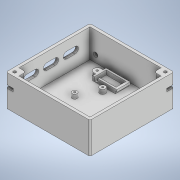
# Autodesk Inventor part: caixa transmissao
Saved by Autodesk Inventor 2022 (Build 260153000, 153)
## iProperties
Created: 2022-03-12
Part Number: caixa transmissao
Material: Genérico
Document SubType Name: Modeling
Designer: Hanter
Density: 1 g/cm^3
Appearance: Padrão
Author: Hanter
Autodesk Inventor part; units mm, degrees
ref_plane "YZ Plane" through (0, 0, 0) normal (1, 0, 0) x (0, 1, 0)
ref_plane "XZ Plane" through (0, 0, 0) normal (0, 1, 0) x (-1, 0, 0)
ref_plane "XY Plane" through (0, 0, 0) normal (0, 0, 1) x (1, 0, 0)
sketch "Esboço1" plane through (0, 0, 0) normal (0, 1, 0) x (-1, 0, 0)
  line L0 (-55, 55) -> (55, 55)
  line L1 (55, 55) -> (55, -55)
  line L2 (55, -55) -> (-55, -55)
  line L3 (-55, -55) -> (-55, 55)
  line L4 (-55, 55) -> (55, -55) construction
  line L5 (55, 55) -> (-55, -55) construction
  point P0 (0, 0)
  dimension "d0" = 110
  dimension "d1" = 110
  constraints: 12 end point, 2 midpoint, 2 parallel, 1 horizontal, 1 perpendicular
  measures "d0" distance of L1.end L2.end
  measures "d1" distance of L0.end L1.end
extrude "Extrusão1" add sketch "Esboço1" along normal blind 3 and the other way blind 1
sketch "Esboço2" plane through (0, 3, 0) normal (0, 1, 0) x (1, 0, 0)
  line L0 (47, -47) -> (-9.07, -47)
  line L1 (47, 26.73) -> (47, -47)
  line L2 (55, -55) -> (55, 55) projected
  line L3 (-55, -55) -> (55, -55) projected
  circle A0 centre (44.23, -44.26) radius 1.35
  circle A1 centre (44.23, 24.32) radius 1.35
  circle A2 centre (-6.57, -44.26) radius 1.35
  circle A3 centre (-6.57, 24.32) radius 1.35
  circle A4 centre (-6.57, -44.26) radius 4
  circle A5 centre (-6.57, 24.32) radius 4
  circle A6 centre (44.23, 24.32) radius 4
  circle A7 centre (44.23, -44.26) radius 4
  point P0 (0, 0)
  dimension "d8" = 2.7
  dimension "d13" = 68.58
  dimension "d16" = 50.8
  dimension "d21" = 8
  dimension "d22" = 8
  dimension "d23" = 8
  dimension "d24" = 8
  constraints: 8 centre point, 4 coincident, 4 end point, 2 horizontal, 1 vertical, 6 other
  measures "d8" diameter of A0
  measures "d13" distance of A0.centre A1.centre
  measures "d16" distance of A0.centre A2.centre
  measures "d21" diameter of A4
  measures "d22" diameter of A5
  measures "d23" diameter of A6
  measures "d24" diameter of A7
extrude "Extrusão2" add sketch "Esboço2" along normal blind 6
sketch "Esboço3" plane through (0, 3, 0) normal (0, 1, 0) x (1, 0, 0)
  line L0 (47, -47) -> (-9.07, -47)
  line L1 (-9.07, -47) -> (-9.07, 26.73)
  line L2 (-9.07, 26.73) -> (47, 26.73)
  line L3 (47, 26.73) -> (47, -47)
  line L4 (55, -55) -> (55, 55) projected
  line L5 (-55, -55) -> (55, -55) projected
  line L6 (55, 55) -> (-55, 55) projected
  line L7 (-55, -55) -> (-55, 55) projected
  circle A0 centre (-36.1, -31.5) radius 1.4
  circle A1 centre (-20.1, -1.5) radius 1.4
  circle A2 centre (-36.1, -31.5) radius 3.5
  circle A3 centre (-20.1, -1.5) radius 3.5
  point P0 (0, 0)
  dimension "d27" = 56.07
  dimension "d28" = 73.73
  dimension "d29" = 8
  dimension "d30" = 8
  dimension "d42" = 2.8
  dimension "d43" = 2.8
  dimension "d49" = 7
  dimension "d50" = 7
  constraints: 8 end point, 4 centre point, 2 coincident, 2 parallel, 1 horizontal, 1 perpendicular
  measures "d27" distance of L1.end L2.end
  measures "d28" distance of L0.end L1.end
  measures "d29" distance between parallel lines of L4 L3
  measures "d30" distance between parallel lines of L5 L0
  measures "d42" diameter of A0
  measures "d43" diameter of A1
  measures "d49" diameter of A2
  measures "d50" diameter of A3
extrude "Extrusão3" add sketch "Esboço3" along normal blind 6 contours A2 | A3
sketch "Esboço4" plane through (0, 3, 0) normal (0, 1, 0) x (1, 0, 0)
  line L0 (47, -47) -> (-9.07, -47)
  line L1 (-9.07, -47) -> (-9.07, 26.73)
  line L2 (-9.07, 26.73) -> (47, 26.73)
  line L3 (47, 26.73) -> (47, -47)
  line L4 (55, -55) -> (55, 55) projected
  line L5 (-55, -55) -> (55, -55) projected
  line L6 (-38.6, -38) -> (-17.6, -38)
  line L7 (-17.6, -38) -> (-17.6, 5)
  line L8 (-17.6, 5) -> (-38.6, 5)
  line L9 (-38.6, 5) -> (-38.6, -38)
  line L10 (-55, 55) -> (-55, -55) projected
  line L11 (3, 47.7) -> (-25, 47.7)
  line L12 (-25, 47.7) -> (-25, 33.7)
  line L13 (-25, 33.7) -> (3, 33.7)
  line L14 (3, 33.7) -> (3, 47.7)
  line L15 (55, 55) -> (-55, 55) projected
  line L16 (-27.5, 31.2) -> (6.5, 31.2)
  line L17 (6.5, 31.2) -> (6.5, 50.2)
  line L18 (6.5, 50.2) -> (-27.5, 50.2)
  line L19 (-27.5, 50.2) -> (-27.5, 31.2)
  line L20 (-27.5, 35.7) -> (-35.5, 35.7)
  line L21 (-35.5, 35.7) -> (-35.5, 45.7)
  line L22 (-35.5, 45.7) -> (-27.5, 45.7)
  line L23 (-27.5, 45.7) -> (-27.5, 35.7)
  point P0 (0, 0)
  dimension "d53" = 56.07
  dimension "d54" = 73.73
  dimension "d55" = 8
  dimension "d56" = 8
  dimension "d57" = 21
  dimension "d58" = 43
  dimension "d59" = 16.4
  dimension "d60" = 17
  dimension "d64" = 52
  dimension "d65" = 14
  dimension "d66" = 28
  dimension "d67" = 2.5
  dimension "d68" = 2.5
  dimension "d69" = 2.5
  dimension "d70" = 3.5
  dimension "d71" = 8
  dimension "d81" = 2
  dimension "d82" = 2
  constraints: 40 end point, 10 parallel, 5 horizontal, 5 perpendicular, 1 point on line
  measures "d53" distance of L1.end L2.end
  measures "d54" distance of L0.end L1.end
  measures "d55" distance between parallel lines of L4 L3
  measures "d56" distance between parallel lines of L5 L0
  measures "d57" distance of L8.end L7.end
  measures "d58" distance of L7.end L6.end
  measures "d59" distance between parallel lines of L10 L9
  measures "d60" distance between parallel lines of L5 L6
  measures "d64" distance between parallel lines of L4 L14
  measures "d65" distance of L11.end L12.end
  measures "d66" distance of L11.start L11.end
  measures "d67" distance between parallel lines of L11 L18
  measures "d68" distance between parallel lines of L16 L13
  measures "d69" distance between parallel lines of L19 L12
  measures "d70" distance between parallel lines of L17 L14
  measures "d71" distance of L21.end L22.end
  measures "d81" distance between parallel lines of L13 L20
  measures "d82" distance between parallel lines of L11 L22
extrude "Extrusão4" add sketch "Esboço4" along normal blind 6 contours L19 L18 L17 L16 | L20 L21 L22 L19
sketch "Esboço5" plane through (-27.5, 3, -31.2) normal (0, 0, 1) x (1, 0, 0)
  line L0 (2.5, 0) -> (2.5, 6) projected
  line L1 (2.5, 6) -> (7.5, 6)
  line L2 (7.5, 6) -> (7.5, 1)
  line L3 (7.5, 1) -> (2.5, 1)
  line L4 (2.5, 1) -> (2.5, 6)
  point P0 (27.5, -3)
  point P1 (2.5, 1)
  dimension "d74" = 5
  dimension "d75" = 5
  constraints: 8 end point, 2 parallel, 1 horizontal, 1 perpendicular
  measures "d74" distance of L2.end L3.end
  measures "d75" distance of L1.end L2.end
extrude "Extrusão5" cut sketch "Esboço5" against normal blind 8
sketch "Esboço6" plane through (0, 9, 0) normal (0, 1, 0) x (1, 0, 0)
  circle A0 centre (-30.5, 40.7) radius 1.45
  line L0 (-35.5, 45.7) -> (-35.5, 35.7) projected
  line L1 (-27.5, 45.7) -> (-35.5, 45.7) projected
  point P0 (0, 0)
  dimension "d78" = 2.9
  dimension "d79" = 5
  dimension "d80" = 5
  constraints: 1 centre point
  measures "d78" diameter of A0
  measures "d79" distance from line of L0 A0.centre
  measures "d80" distance from line of L1 A0.centre
extrude "Extrusão6" cut sketch "Esboço6" against normal blind 7
fillet "Arredondamento1" radius 5 2 edges at (-35.5, 6, -45.7) (-35.5, 6, -35.7)
sketch "Esboço10" plane through (6.5, 3, -31.2) normal (1, 0, 0) x (0, 0, -1)
  line L0 (0, 0) -> (0, 6) projected
  line L1 (19, 0) -> (19, 6) projected
  line L2 (0, 0) -> (19, 0)
  line L3 (19, 0) -> (19, 2.8)
  line L4 (19, 2.8) -> (0, 2.8)
  line L5 (0, 2.8) -> (0, 0)
  point P0 (-31.2, -3)
  point P1 (0, 2.8)
  dimension "d95" = 2.8
  constraints: 8 end point, 2 parallel, 1 horizontal, 1 perpendicular, 1 point on line
  measures "d95" distance of L3.end L2.end
extrude "Extrusão9" cut sketch "Esboço10" against normal blind 2
sketch "Esboço11" plane through (0, 3, 0) normal (0, 1, 0) x (1, 0, 0)
  line L0 (-55, -55) -> (55, -55) projected
  line L1 (55, 55) -> (-55, 55)
  line L2 (-55, 55) -> (-55, -55)
  line L3 (-55, -55) -> (55, -55)
  line L4 (55, -55) -> (55, 55)
  line L5 (59, -59) -> (-59, -59)
  line L6 (-59, -59) -> (-59, 59)
  line L7 (-59, 59) -> (59, 59)
  line L8 (59, 59) -> (59, -59)
  line L9 (59, -59) -> (-59, 59) construction
  line L10 (-59, -59) -> (59, 59) construction
  point P0 (0, 0)
  dimension "d98" = 118
  dimension "d99" = 118
  constraints: 20 end point, 4 parallel, 2 horizontal, 2 midpoint, 2 perpendicular
  measures "d98" distance of L6.end L7.end
  measures "d99" distance of L5.end L6.end
extrude "Extrusão10" add sketch "Esboço11" along normal blind 40 and the other way blind 4
sketch "Esboço12" plane through (-59, -1, 59) normal (-1, 0, 0) x (0, 0, 1)
  arc A0 (-25, 21.35) -> (-25, 30.65) centre (-25, 26) ccw
  line L0 (0, 0) -> (0, 44) projected
  arc A1 (-37, 30.65) -> (-37, 21.35) centre (-37, 26) ccw
  arc A2 (-53, 21.35) -> (-53, 30.65) centre (-53, 26) ccw
  arc A3 (-65, 30.65) -> (-65, 21.35) centre (-65, 26) ccw
  arc A4 (-81, 21.35) -> (-81, 30.65) centre (-81, 26) ccw
  arc A5 (-93, 30.65) -> (-93, 21.35) centre (-93, 26) ccw
  line L1 (-93, 30.65) -> (-81, 30.65)
  line L2 (-81, 21.35) -> (-93, 21.35)
  line L3 (-65, 30.65) -> (-53, 30.65)
  line L4 (-53, 21.35) -> (-65, 21.35)
  line L5 (-37, 30.65) -> (-25, 30.65)
  line L6 (-25, 21.35) -> (-37, 21.35)
  line L7 (0, 0) -> (-118, 0) projected
  point P0 (-59, 1)
  dimension "d106" = 9.3
  dimension "d107" = 25
  dimension "d108" = 9.3
  dimension "d109" = 12
  dimension "d110" = 9.3
  dimension "d111" = 9.3
  dimension "d112" = 16
  dimension "d113" = 12
  dimension "d114" = 9.3
  dimension "d115" = 16
  dimension "d116" = 9.3
  dimension "d117" = 12
  dimension "d120" = 26
  dimension "d121" = 26
  dimension "d122" = 26
  dimension "d123" = 26
  dimension "d124" = 26
  dimension "d125" = 26
  constraints: 12 end point, 12 point on circle, 8 point on line, 6 centre point, 3 tangent
  measures "d106" diameter of A0
  measures "d107" distance from line of L0 A0.centre
  measures "d108" diameter of A1
  measures "d109" distance of A0.centre A1.centre
  measures "d110" diameter of A2
  measures "d111" diameter of A3
  measures "d112" distance of A1.centre A2.centre
  measures "d113" distance of A2.centre A3.centre
  measures "d114" diameter of A4
  measures "d115" distance of A3.centre A4.centre
  measures "d116" diameter of A5
  measures "d117" distance of A4.centre A5.centre
  measures "d120" distance from line of L7 A0.centre
  measures "d121" distance from line of L7 A1.centre
  measures "d122" distance from line of L7 A2.centre
  measures "d123" distance from line of L7 A3.centre
  measures "d124" distance from line of L7 A4.centre
  measures "d125" distance from line of L7 A5.centre
extrude "Extrusão11" cut sketch "Esboço12" against normal blind 40
sketch "Esboço13" plane through (59, 43, -59) normal (0, 0, -1) x (-1, 0, 0)
  circle A0 centre (106, -30) radius 3.125
  line L0 (118, -44) -> (0, -44) projected
  line L1 (118, -44) -> (118, 0) projected
  point P0 (59, -43)
  dimension "d126" = 6.25
  dimension "d127" = 14
  dimension "d128" = 12
  constraints: 1 centre point
  measures "d126" diameter of A0
  measures "d127" distance from line of L0 A0.centre
  measures "d128" distance from line of L1 A0.centre
extrude "Extrusão12" cut sketch "Esboço13" against normal blind 40
sketch "Esboço14" plane through (0, 43, 0) normal (0, 1, 0) x (1, 0, 0)
  line L0 (-55, 55) -> (55, 55) projected
  line L1 (55, 55) -> (45, 55)
  line L2 (45, 55) -> (45, 45)
  line L3 (45, 45) -> (55, 45)
  line L4 (55, 45) -> (55, 55)
  line L5 (-55, 55) -> (-55, -55) projected
  line L6 (-55, -55) -> (-45, -55)
  line L7 (-45, -55) -> (-45, -45)
  line L8 (-45, -45) -> (-55, -45)
  line L9 (-55, -45) -> (-55, -55)
  point P0 (0, 0)
  dimension "d131" = 10
  dimension "d132" = 10
  dimension "d133" = 10
  dimension "d134" = 10
  constraints: 16 end point, 4 parallel, 2 horizontal, 2 perpendicular
  measures "d131" distance of L3.end L2.end
  measures "d132" distance of L2.end L1.end
  measures "d133" distance of L8.end L7.end
  measures "d134" distance of L7.end L6.end
extrude "Extrusão13" add sketch "Esboço14" against normal blind 40
fillet "Arredondamento2" radius 2 4 edges at (-59, 21, 59) (59, 21, 59) (59, 21, -59) (-59, 21, -59)
fillet "Arredondamento3" radius 4 2 edges at (45, 23, -45) (-45, 23, 45)
sketch "Esboço15" plane through (-59, -1, -57) normal (-1, 0, 0) x (0, 0, 1)
  line L0 (116, 44) -> (116, 0) projected
  line L1 (116, 29) -> (106, 29)
  line L2 (106, 29) -> (106, 25)
  line L3 (106, 25) -> (116, 25)
  line L4 (116, 25) -> (116, 29)
  line L5 (0, 44) -> (114, 44) projected
  point P0 (57, 1)
  dimension "d139" = 10
  dimension "d140" = 4
  dimension "d141" = 15
  constraints: 8 end point, 2 parallel, 1 horizontal, 1 perpendicular, 1 point on line
  measures "d139" distance of L3.end L2.end
  measures "d140" distance of L2.end L1.end
  measures "d141" distance between parallel lines of L5 L1
extrude "Extrusão14" cut sketch "Esboço15" against normal blind 10
sketch "Esboço16" plane through (59, -1, -57) normal (1, 0, 0) x (0, 0, -1)
  line L0 (2, 44) -> (2, 0) projected
  line L1 (2, 29) -> (-8, 29)
  line L2 (-8, 29) -> (-8, 25)
  line L3 (-8, 25) -> (2, 25)
  line L4 (2, 25) -> (2, 29)
  line L5 (-114, 44) -> (0, 44) projected
  point P0 (-57, 1)
  point P1 (2, 25)
  dimension "d144" = 10
  dimension "d145" = 4
  dimension "d148" = 15
  constraints: 8 end point, 2 parallel, 1 horizontal, 1 perpendicular, 1 point on line
  measures "d144" distance of L3.end L2.end
  measures "d145" distance of L2.end L1.end
  measures "d148" distance between parallel lines of L1 L5
extrude "Extrusão15" cut sketch "Esboço16" against normal blind 10
sketch "Esboço17" plane through (0, 43, 0) normal (0, 1, 0) x (1, 0, 0)
  circle A0 centre (-53, -53) radius 2.005
  line L0 (-57, -59) -> (57, -59) projected
  line L1 (-59, 57) -> (-59, -57) projected
  circle A1 centre (53, 53) radius 2.005
  line L2 (59, -57) -> (59, 57) projected
  line L3 (57, 59) -> (-57, 59) projected
  point P0 (0, 0)
  dimension "d149" = 4.01
  dimension "d150" = 6
  dimension "d151" = 6
  dimension "d152" = 4.01
  dimension "d153" = 6
  dimension "d154" = 6
  constraints: 2 centre point
  measures "d149" diameter of A0
  measures "d150" distance from line of L0 A0.centre
  measures "d151" distance from line of L1 A0.centre
  measures "d152" diameter of A1
  measures "d153" distance from line of L2 A1.centre
  measures "d154" distance from line of L3 A1.centre
extrude "Extrusão16" cut sketch "Esboço17" against normal blind 32
sketch "Esboço21" plane through (0, 3, 0) normal (0, 1, 0) x (1, 0, 0)
  circle A0 centre (18.5, 43) radius 3
  line L0 (6.5, 31.2) -> (6.5, 50.2) projected
  line L1 (-55, 55) -> (45, 55) projected
  circle A1 centre (18.5, -43) radius 3
  line L2 (55, -55) -> (-45, -55) projected
  point P0 (0, 0)
  dimension "d174" = 6
  dimension "d175" = 12
  dimension "d176" = 12
  dimension "d177" = 6
  dimension "d178" = 12
  dimension "d181" = 86
  constraints: 2 centre point
  measures "d174" diameter of A0
  measures "d175" distance from line of L0 A0.centre
  measures "d176" distance from line of L1 A0.centre
  measures "d177" diameter of A1
  measures "d178" distance from line of L2 A1.centre
  measures "d181" distance of A0.centre A1.centre
extrude "Extrusão18" cut sketch "Esboço21" against normal blind 10
